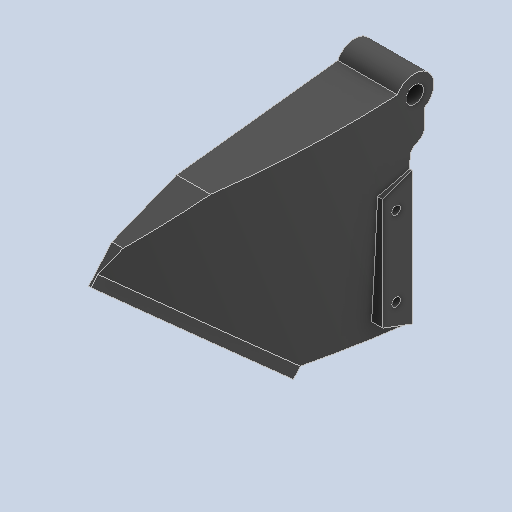
# Autodesk Inventor part: chest_base_right
Saved by Autodesk Inventor 2026.1 (Build 301233020, 233B)
## iProperties
Created: 2024-10-10
Part Number: chest_base_right
Material: 一般
Document SubType Name: Modeling
Designer: hibik
Density: 1 g/cm^3
Appearance: 既定
Author: hibik
Autodesk Inventor part; units mm, degrees
ref_plane "YZ Plane" through (0, 0, 0) normal (1, 0, 0) x (0, 1, 0)
ref_plane "XZ Plane" through (0, 0, 0) normal (0, 1, 0) x (-1, 0, 0)
ref_plane "XY Plane" through (0, 0, 0) normal (0, 0, 1) x (1, 0, 0)
sketch "スケッチ1" plane through (0, 0, 0) normal (1, 0, 0) x (0, 1, 0)
  line L0 (0, 0) -> (27, 0)
  line L1 (27, 0) -> (27, 50)
  line L2 (27, 50) -> (0, 50)
  line L3 (0, 50) -> (0, 0)
  line L4 (27, 50) -> (0, 19)
  arc A0 (46.7739, 0) -> (27, 50) centre (-26.3276, 0) ccw construction
  line L5 (46.7739, 0) -> (46.7739, 12.8727) construction
  line L6 (27, 0) -> (46.7739, 0)
  circle A1 centre (21, 5.5) radius 0.8
  circle A2 centre (6, 5.5) radius 0.8
  line L7 (27, 50) -> (29.2187, 52.5474)
  line L8 (46.7739, 0) -> (19.4069, 0)
  line L9 (27, 50) -> (46.7739, 0) construction
  line L10 (29.2187, 52.5474) -> (50, 0)
  line L11 (46.7739, 0) -> (50, 0)
  dimension "d0" = 27
  dimension "d1" = 50
  dimension "d7" = 1.6
  dimension "d8" = 5.5
  dimension "d9" = 6
  dimension "d10" = 6
  dimension "d24" = 3
  dimension "d58" = 23
  dimension "d59" = 19
  constraints: 24 end point, 3 centre point, 3 horizontal, 3 horizontal alignment, 3 parallel, 2 point on circle, 2 point on line, 1 collinear, 1 equal radius, 1 perpendicular, 1 tangent, 1 vertical
  measures "d0" distance of L2.end L1.end
  measures "d1" distance of L1.end L0.end
  measures "d7" diameter of A1
  measures "d8" distance from line of L0 A1.centre
  measures "d9" distance from line of L1 A1.centre
  measures "d10" distance from line of L3 A2.centre
  measures "d24" distance between parallel lines of L9 L10
  measures "d58" distance of L0.end L10.end
  measures "d59" distance of L0.start L4.end
extrude "押し出し1" add sketch "スケッチ1" along normal blind 11.5 contours L3 L4 L1 L0 | L1 L7 L10 L11 L6
sketch "スケッチ7" plane through (0, 29.2187, 52.5474) normal (0, 0.9299196, 0.367763) x (1, 0, 0)
  line L0 (11.5, 38.1193) -> (11.5, 56.5074) projected
  arc A0 (0, 0) -> (11.5, 56.5074) centre (-133.0799, 56.5074) ccw
  line L1 (11.5, 56.5074) -> (11.5, 0) projected
  line L2 (0, 0) -> (11.5, 0) projected
  point P0 (0, 38.1193)
  constraints: 2 point on circle, 1 centre point, 1 tangent
extrude "押し出し5" cut sketch "スケッチ7" against normal through all
sketch "スケッチ8" plane through (0, 0, 0) normal (-1, 0, 0) x (0, 0, 1)
  line L0 (0, 0) -> (8, 3)
  line L1 (8, 3) -> (8, 24)
  line L2 (8, 24) -> (0, 27)
  circle A0 centre (5.5, 21) radius 0.8 projected
  line L3 (0, 0) -> (0, 50) projected
  circle A1 centre (5.5, 6) radius 0.8 projected
  dimension "d28" = 3
  dimension "d29" = 3
  dimension "d30" = 8
  dimension "d31" = 3
  constraints: 6 end point, 1 point on line, 1 vertical
  measures "d28" vertical distance of L0.start L0.end
  measures "d29" vertical distance of L1.end A0.centre
  measures "d30" distance between parallel lines of L3 L1
  measures "d31" vertical distance of L1.end L2.end
extrude "押し出し6" add sketch "スケッチ8" against normal up to surface (11.5 mm away)
sketch "スケッチ9" plane through (0, 0, 0) normal (-1, 0, 0) x (0, 0, 1)
  line L0 (0, 50) -> (52.5474, 29.2187) projected
  line L1 (0, 0) -> (0, 50) projected
  line L2 (0, 40.082) -> (35.4002, 36)
  dimension "d37" = 14
  dimension "d38" = 15
  constraints: 2 end point, 2 point on line
  measures "d37" vertical distance of L0.start L2.end
  measures "d38" angle of L0 L2
extrude "押し出し7" cut sketch "スケッチ9" against normal through all
sketch "スケッチ10" plane through (0, 0, 0) normal (-1, 0, 0) x (0, 0, 1)
  circle A0 centre (1.85, 38.0064) radius 1.85
  line L0 (35.4002, 36) -> (0, 40.082) projected
  line L1 (0, 0) -> (0, 40.082) projected
  circle A1 centre (1.85, 38.0064) radius 1.6
  dimension "d39" = 3.2
  dimension "d40" = 3.7
  constraints: 2 centre point, 2 tangent, 1 coincident
  measures "d39" diameter of A1
  measures "d40" diameter of A0
extrude "押し出し8" cut sketch "スケッチ10" against normal through all contours A1
sketch "スケッチ11" plane through (0, 0, 0) normal (-1, 0, 0) x (0, 0, 1)
  circle A0 centre (1.85, 38.0064) radius 1.6 projected
  circle A1 centre (1.85, 38.0064) radius 3.5
  point P0 (0, 0)
  dimension "d43" = 7
  constraints: 1 centre point, 1 coincident
  measures "d43" diameter of A1
extrude "押し出し9" add sketch "スケッチ11" against normal up to surface round surface about axis through (-133.0799, 50, 0) along (0, -0.9299196, -0.367763) radius 144.5799 far side no
sketch "スケッチ12" plane through (0, 0, 0) normal (-1, 0, 0) x (0, 0, 1)
  line L0 (0, 0) -> (2.5, 0)
  line L1 (2.5, 0) -> (2.5, 30)
  line L2 (2.5, 30) -> (0, 30)
  line L3 (0, 30) -> (0, 0)
  dimension "d47" = 2.5
  dimension "d48" = 30
  constraints: 8 end point, 2 parallel, 1 horizontal, 1 perpendicular
  measures "d47" distance of L2.end L1.end
  measures "d48" distance of L1.end L0.end
extrude "押し出し10" cut sketch "スケッチ12" against normal through all
fillet "フィレット3" radius 2 2 edges at (5.5878, 30, 2.5) (5.6564, 30, 0)
sketch "スケッチ13" plane through (0, 0, 0) normal (-1, 0, 0) x (0, 0, 1)
  line L0 (2.5, 28) -> (2.5, 0) projected
  line L1 (19, 0) -> (2.5, 0) projected
  circle A0 centre (5.5, 21) radius 0.8 projected
  circle A1 centre (5.5, 6) radius 0.8 projected
  line L2 (39.4201, 28.3942) -> (6.8194, 0)
  line L3 (52.5474, 29.2187) -> (19, 0) projected
  line L4 (4.4341, 30.7455) -> (38.7284, 17.1828)
  line L5 (35.4002, 36) -> (52.5474, 29.2187) projected
  line L6 (1.85, 38.0064) -> (33.512, 34.3555)
  line L7 (4.8196, 36.154) -> (31.9811, 33.0221)
  line L8 (35.4002, 36) -> (21.5812, 23.9641)
  circle A2 centre (1.85, 38.0064) radius 3.5
  arc A3 (0, 31.7081) -> (1.25, 29.854) centre (2, 31.7081) ccw projected
  arc A4 (2.5, 28) -> (1.25, 29.854) centre (0.5, 28) ccw projected
  line L9 (52.5474, 29.2187) -> (19, 0) projected
  line L10 (35.4002, 36) -> (52.5474, 29.2187) projected
  line L11 (35.4002, 36) -> (5.0135, 39.5039) projected
  arc A5 (5.0135, 39.5039) -> (0, 35.0353) centre (1.85, 38.0064) ccw projected
  line L12 (0, 31.7081) -> (0, 35.0353) projected
  arc A6 (5.0135, 39.5039) -> (0, 35.0353) centre (1.85, 38.0064) ccw projected
  line L13 (35.4002, 36) -> (5.0135, 39.5039) projected
  point P0 (0, 0)
  point P1 (30.3515, 20.4957)
  point P2 (27.5488, 14.4588)
  point P3 (40.9181, 19.0899)
  dimension "d56" = 1.5
  dimension "d60" = 8
  constraints: 10 end point, 6 point on line, 4 parallel, 1 coincident, 1 midpoint, 7 other
  measures "d56" distance between parallel lines of L6 L7
  measures "d60" distance between parallel lines of L3 L2
extrude "押し出し11" add sketch "スケッチ13" along normal blind 2 contours A4 A3 L12 A2 L7 L8 L4 L2 L1 L0
sketch "スケッチ14" plane through (0, 0, 19) normal (0, -0.7540816, 0.6567807) x (1, 0, 0)
  ellipse E0 centre (-133.0799, -78.4359) end of major axis (-133.0799, -392.9482) minor radius 144.5799 (6.9318, 0) -> (0, 44.4877) ccw projected
  ellipse E1 centre (-133.0799, -78.4359) end of major axis (-133.0799, -392.9482) minor radius 144.5799 (6.9318, 0) -> (0, 44.4877) ccw projected
  line L0 (0, 44.4877) -> (0, 0) projected
  line L1 (0, 0) -> (6.9318, 0) projected
  point P0 (0, -14.3276)
  point P1 (6.9318, 0)
  point P2 (0, 44.4877)
  constraints: 2 other
extrude "押し出し12" add sketch "スケッチ14" along normal blind 2
sketch "スケッチ15" plane through (0, -1.5082, 20.3136) normal (0, -0.7540816, 0.6567807) x (1, 0, 0)
  line L0 (-42, 42.0573) -> (-33, 42.0573) projected
  line L1 (0, 44.4877) -> (0, 0) projected
  ellipse E0 centre (-133.0799, -78.4359) end of major axis (-133.0799, -392.9482) minor radius 144.5799 (6.9318, 0) -> (0, 44.4877) ccw projected
  line L2 (-33, 42.0573) -> (2.123, 42.0573)
  ellipse E1 centre (-133.0799, 18.5115) end of major axis (-277.6599, 18.5115) minor radius 66.4628 (6.3983, 36.0112) -> (0, 44.4877) ccw projected
  point P0 (0, -14.3276)
  point P1 (0, 42.0573)
  constraints: 2 end point, 1 horizontal, 3 other
extrude "押し出し13" cut sketch "スケッチ15" against normal through all
equation "\"d10\" = d9"
equation "\"d29\" = d28"
